Autodesk Fusion 360 part; units mm, degrees
(part 25 of 25)
sketch "Sketch1 (2)" plane through (150, 0, 0) normal (1, 0, 0) x (0, 1, 0) in component "RIght"
  line L0 (64, 0) -> (80, 0)
  line L1 (80, 0) -> (80, 3)
  line L2 (80, 3) -> (64, 3) construction
  line L3 (0, 3) -> (0, 0)
  line L4 (0, 3) -> (0, 160)
  line L5 (0, 160) -> (83, 112.0799)
  line L6 (80, 3) -> (80, 108.0799)
  line L7 (80, 108.0799) -> (83, 108.0799)
  line L8 (83, 108.0799) -> (83, 112.0799)
  circle A0 centre (5.9574, 158.3503) radius 2.9841
  line L9 (4.524, 160.9676) -> (8.9408, 158.4176) construction
  line L10 (8.9408, 158.4176) -> (7.3908, 155.7329) construction
  line L11 (7.3908, 155.7329) -> (2.974, 158.2829) construction
  line L12 (2.974, 158.2829) -> (4.524, 160.9676) construction
  arc A1 (11.1398, 155.3582) -> (0, 157.7854) centre (5.9574, 158.3503) ccw
  line L13 (-5.009, 151.3242) -> (0, 160) construction
  line L14 (11.1398, 155.3582) -> (10.3648, 154.0159) construction
  arc A2 (11.1398, 155.3582) -> (11.7071, 153.2409) centre (12.4821, 154.5832) ccw
  line L15 (64, 3) -> (64, 0)
  line L16 (0, 0) -> (16, 0)
  line L17 (16, 0) -> (16, 3)
  line L18 (80, 0) -> (80, 3)
  line L19 (64, 0) -> (80, 0)
  line L20 (64, 0) -> (64, 3)
  line L21 (48, 3) -> (64, 3)
  line L22 (48, 0) -> (48, 3)
  line L23 (32, 0) -> (48, 0)
  line L24 (32, 0) -> (32, 3)
  line L25 (16, 3) -> (32, 3)
  line L26 (57.0192, 127.0799) -> (58.5192, 129.678)
  line L27 (58.5192, 129.678) -> (67.1795, 124.678)
  line L28 (67.1795, 124.678) -> (65.6795, 122.0799)
  line L29 (0, 145) -> (3, 145)
  line L30 (3, 145) -> (3, 130)
  line L31 (3, 130) -> (0, 130)
  line L32 (80, 68.04) -> (83, 68.04)
  line L33 (83, 68.04) -> (83, 43.04)
  line L34 (83, 43.04) -> (80, 43.04)
  line L35 (83, 55.54) -> (80, 55.54) construction
  dimension "d13" = 60
  dimension "d14" = 160
  dimension "d22" = 3
  dimension "d23" = 4
  dimension "d24" = 3.1
  dimension "d25" = 5.1
  dimension "d26" = 3
  dimension "d45" = 3
  dimension "d46" = 10
  dimension "d47" = 20
  dimension "d54" = 3
  dimension "d55" = 15
  dimension "d56" = 15
  dimension "d60" = 25
  constraint perpendicular L2 L4
  constraint coincident L1.end L2.start
  constraint perpendicular L2 L6
  constraint perpendicular L6 L7
  constraint perpendicular L7 L8
  constraint perpendicular L9 L10
  constraint parallel L9 L11
  constraint parallel L10 L12
  constraint coincident A0 L9.end
  constraint coincident A0 L9.start
  constraint coincident A0 L10.end
  constraint collinear L5 L11
  constraint coincident A0.centre A1.centre
  constraint coincident L5 L14.end
  constraint tangent A1 L14
  constraint perpendicular L5 L13
  constraint perpendicular L5 L14
  constraint tangent A1 L13
  constraint coincident L4 A1.end
  constraint tangent A1 A2
  constraint tangent L5 A2
  constraint coincident L5 A2.end
  constraint coincident L3.start L4.start
  constraint coincident L5 L26.start
  constraint perpendicular L5 L26
  constraint perpendicular L26 L27
  constraint coincident L5 L28.end
  constraint perpendicular L5 L28
  constraint coincident L4 L29.start
  constraint perpendicular L4 L29
  constraint perpendicular L29 L30
  constraint coincident L4 L31.end
  constraint perpendicular L4 L31
  constraint coincident L6 L32.start
  constraint perpendicular L6 L32
  constraint perpendicular L32 L33
  constraint coincident L6 L34.end
  constraint perpendicular L6 L34
  constraint collinear L8 L33
  constraint midpoint L33 L35.start
  constraint midpoint L6 L35.end
  constraint perpendicular L33 L35
  measures "d13" angle of L4 L5
  measures "d14" distance of L3.end L4.end
  measures "d22" distance of L6.end L7.end
  measures "d23" distance of L5.end L7.end
  measures "d24" distance of L9.end L10.end
  measures "d25" distance of L9.start L9.end
  measures "d26" distance of A0 A1
  measures "d45" distance of L26.start L26.end
  measures "d46" distance of L26.end L27.end
  measures "d47" distance of L5.end L28
  measures "d54" distance of L29.start L29.end
  measures "d55" distance of L29.end L30.end
  measures "d56" distance of L4.end L29
  measures "d60" distance of L32.end L33.end
extrude "Extrude1'" add sketch "Sketch1 (2)" along normal blind 3 separate body contours L0 L1 L3 L4 L5 L6 L7 L8 A0 A1 L15 L16 L17 L18 L19 L20 L21 L22 L23 L24 L25 L29 L30 L31 | L6 L32 L33 L34 | L5 L26 L27 L28 | L5 A0 A1 A2 makes body 2 in component "RIght"
sketch "Sketch1 (3)" plane through (0, 0, 0) normal (-1, 0, 0) x (0, -1, 0) in component "Left"
  arc A0 (0, 158.9152) -> (-11.1398, 155.3582) centre (-5.9574, 158.3503) ccw
  arc A1 (-11.7071, 153.2409) -> (-11.1398, 155.3582) centre (-12.4821, 154.5832) ccw
  line L0 (-11.7071, 153.2409) -> (-57.0192, 127.0799)
  circle A2 centre (-5.9574, 158.3503) radius 2.9841
  line L1 (0, 145) -> (0, 158.9152)
  line L2 (-83, 112.0799) -> (-83, 108.0799)
  line L3 (-83, 108.0799) -> (-80, 108.0799)
  line L4 (-80, 43.04) -> (-80, 0)
  line L5 (-80, 0) -> (-64, 0)
  line L6 (-64, 0) -> (-64, 3)
  line L7 (-64, 3) -> (-48, 3)
  line L8 (-48, 3) -> (-48, 0)
  line L9 (-48, 0) -> (-32, 0)
  line L10 (-32, 0) -> (-32, 3)
  line L11 (-32, 3) -> (-16, 3)
  line L12 (-16, 3) -> (-16, 0)
  line L13 (-16, 0) -> (0, 0)
  line L14 (-57.0192, 127.0799) -> (-58.5192, 129.678)
  line L15 (-58.5192, 129.678) -> (-67.1795, 124.678)
  line L16 (-67.1795, 124.678) -> (-65.6795, 122.0799)
  line L17 (-65.6795, 122.0799) -> (-83, 112.0799)
  line L18 (-3, 145) -> (0, 145)
  line L19 (0, 0) -> (0, 130)
  line L20 (0, 130) -> (-3, 130)
  line L21 (-3, 130) -> (-3, 145)
  line L22 (-80, 108.0799) -> (-80, 68.04)
  line L23 (-80, 68.04) -> (-83, 68.04)
  line L24 (-83, 68.04) -> (-83, 43.04)
  line L25 (-83, 43.04) -> (-80, 43.04)
  line L26 (-72.6242, 33.874) -> (-72.6242, 17.226) construction
  line L27 (-72.6242, 17.226) -> (-71.1242, 17.226) construction
  line L28 (-71.1242, 17.226) -> (-71.1242, 33.874) construction
  line L29 (-71.1242, 33.874) -> (-72.6242, 33.874) construction
  line L30 (-74.6242, 35.874) -> (-74.6242, 15.226)
  line L31 (-74.6242, 15.226) -> (-69.1242, 15.226)
  line L32 (-69.1242, 15.226) -> (-69.1242, 35.874)
  line L33 (-69.1242, 35.874) -> (-74.6242, 35.874)
  dimension "d158" = 2
extrude "Extrude1''" add sketch "Sketch1 (3)" along normal blind 3 separate body makes body 3 in component "Left"
sketch "Sketch3" plane through (0, 80, 0) normal (0, 1, 0) x (-1, 0, 0) in component "Back"
  line L0 (-153, 0) -> (-153, 43.04)
  line L1 (3, 43.04) -> (3, 0)
  line L2 (0, 112.0799) -> (0, 108.0799)
  line L3 (-150, 108.0799) -> (-150, 112.0799)
  line L4 (3, 0) -> (-153, 0)
  line L5 (-150, 112.0799) -> (0, 112.0799)
  line L6 (-128.5714, 0) -> (-107.1429, 0)
  line L7 (-107.1429, 0) -> (-107.1429, 3)
  line L8 (-107.1429, 3) -> (-128.5714, 3)
  line L9 (-128.5714, 3) -> (-128.5714, 0)
  line L10 (-85.7143, 0) -> (-64.2857, 0)
  line L11 (-64.2857, 0) -> (-64.2857, 3)
  line L12 (-64.2857, 3) -> (-85.7143, 3)
  line L13 (-85.7143, 3) -> (-85.7143, 0)
  line L14 (-42.8571, 0) -> (-21.4286, 0)
  line L15 (-21.4286, 0) -> (-21.4286, 3)
  line L16 (-21.4286, 3) -> (-42.8571, 3)
  line L17 (-42.8571, 3) -> (-42.8571, 0)
  line L18 (-150, 43.04) -> (-153, 43.04)
  line L19 (-150, 68.04) -> (-150, 43.04)
  line L20 (-150, 68.04) -> (-153, 68.04)
  line L21 (-153, 68.04) -> (-153, 108.0799)
  line L22 (-150, 108.0799) -> (-153, 108.0799)
  line L23 (0, 108.0799) -> (3, 108.0799)
  line L24 (3, 108.0799) -> (3, 68.04)
  line L25 (0, 68.04) -> (3, 68.04)
  line L26 (0, 68.04) -> (0, 43.04)
  line L27 (0, 43.04) -> (3, 43.04)
  circle A0 centre (-6.4309, 71.143) radius 1.5875
  circle A1 centre (-82.7579, 71.143) radius 1.5875
  circle A2 centre (-6.4309, 10.818) radius 1.5875
  circle A3 centre (-82.7579, 10.818) radius 1.5875
  constraint coincident L1.end L4.start
  constraint coincident L0.start L4.end
  constraint coincident L3.end L5.start
  constraint coincident L2.start L5.end
  constraint vertical A1.centre A3.centre
  constraint horizontal A2.centre A3.centre
  constraint equal A0 A3
extrude "Extrude2" add sketch "Sketch3" along normal blind 3 separate body contours L0 L1 L2 L3 L4 L5 L7 L8 L9 L11 L12 L13 L15 L16 L17 L18 L19 L20 L21 L22 L23 L24 L25 L26 L27 makes body 4 in component "Back"
sketch "Sketch1 (4)" plane through (0, 69.282, 120) normal (0, 0.5, 0.866025) x (-1, 0, 0) in component "Fixed Roof"
  line L0 (-150, 4.1599) -> (-153, 4.1599)
  line L1 (-153, 4.1599) -> (-153, -15.8401)
  line L2 (3, 4.1599) -> (3, -15.8401)
  line L3 (0, 4.1599) -> (3, 4.1599)
  line L4 (0, 14.1599) -> (0, 4.1599)
  line L5 (-150, 14.1599) -> (-150, 4.1599)
  line L6 (0, 14.1599) -> (-150, 14.1599)
  line L7 (3, -15.8401) -> (-153, -15.8401)
  constraint coincident L4.start L6.start
  constraint coincident L5.start L6.end
  constraint coincident L2.end L7.start
  constraint coincident L1.end L7.end
extrude "Extrude1'''" add sketch "Sketch1 (4)" along normal blind 3 separate body makes body 5 in component "Fixed Roof"
sketch "Sketch1 (5)" plane through (0, 69.282, 120) normal (0, 0.5, 0.866025) x (-1, 0, 0) in component "Hinged Roof"
  line L0 (-153, 66.4818) -> (-153, 14.1599)
  line L1 (-153, 71.0318) -> (-153, 77)
  line L2 (3, 77) -> (3, 71.0318)
  line L3 (3, 15.1599) -> (-153, 15.1599)
  line L4 (-150, 66.4818) -> (-153, 66.4818)
  line L5 (3, 76.5159) -> (-0.2, 76.5159)
  line L6 (3, 71.5159) -> (-0.2, 71.5159)
  line L7 (-0.2, 76.5159) -> (-0.2, 71.5159) construction
  line L8 (-0.2, 74.0159) -> (3, 74.0159) construction
  line L9 (-0.2, 71.5159) -> (-0.2, 66.4818)
  line L10 (3, 66.4818) -> (-0.2, 66.4818)
  line L11 (0, 77) -> (0, 71.0318) construction
  line L12 (-0.2, 76.5159) -> (-0.2, 78.5159)
  line L13 (-0.2, 78.5159) -> (-149.8, 78.5159)
  line L14 (-75, 15.1599) -> (-75, 78.5159) construction
  line L15 (-153, 66.4818) -> (-149.8, 66.4818)
  line L16 (-149.8, 71.5159) -> (-149.8, 66.4818)
  line L17 (-153, 71.5159) -> (-149.8, 71.5159)
  line L18 (-153, 77) -> (-153, 71.0318)
  line L19 (-153, 76.5159) -> (-149.8, 76.5159)
  line L20 (-149.8, 76.5159) -> (-149.8, 78.5159)
  line L21 (3, 66.4818) -> (3, 14.1599)
  line L22 (-153, 14.1599) -> (-150, 14.1599)
  line L23 (-150, -15.8401) -> (-150, 4.1599)
  line L24 (-150, 4.1599) -> (-153, 4.1599)
  line L25 (-153, 4.1599) -> (-153, -15.8401)
  line L26 (0, 14.1599) -> (-150, 14.1599)
  dimension "d29" = 5
  dimension "d30" = 0.2
  dimension "d31" = 2
  dimension "d34" = 1
  constraint coincident L3.start L21
  constraint coincident L0 L3.end
  constraint perpendicular L0 L3
  constraint coincident L2 L5.start
  constraint perpendicular L2 L5
  constraint coincident L2 L6.start
  constraint perpendicular L2 L6
  constraint midpoint L7 L8.start
  constraint midpoint L2 L8.end
  constraint perpendicular L2 L8
  constraint perpendicular L7 L8
  constraint perpendicular L6 L9
  constraint coincident L10.start L21.start
  constraint perpendicular L9 L10
  constraint perpendicular L5 L12
  constraint perpendicular L12 L13
  constraint midpoint L3 L14.start
  constraint coincident L13 L14.end
  constraint perpendicular L13 L14
  constraint symmetric L2.start L14 L1.end
  constraint symmetric L2.end L14 L1.start
  constraint symmetric L5.start L14 L19.start
  constraint symmetric L5.end L14 L19.end
  constraint symmetric L6.start L14 L17.start
  constraint symmetric L6.end L14 L16.start
  constraint symmetric L9.end L14 L15.end
  constraint symmetric L10.start L14 L0.start
  constraint symmetric L12.end L14 L13.end
  constraint coincident L13.end L20.end
  measures "d29" distance of L5 L6
  measures "d30" distance of L7 L11
  measures "d31" distance of L5.end L12.end
  measures "d34" distance of L3 L26
extrude "Extrude1''''" add sketch "Sketch1 (5)" along normal blind 3 separate body makes body 6 in component "Hinged Roof"
sketch "Sketch4" plane through (0, 3, 0) normal (0, -1, 0) x (1, 0, 0) in component "Front Brace"
  line L0 (0, 130) -> (0, 145)
  line L1 (0, 145) -> (-3, 145)
  line L2 (-3, 145) -> (-3, 130)
  line L3 (-3, 130) -> (0, 130)
  line L4 (150, 145) -> (150, 130)
  line L5 (150, 130) -> (153, 130)
  line L6 (153, 130) -> (153, 145)
  line L7 (153, 145) -> (150, 145)
  line L8 (0, 145) -> (0, 147.5)
  line L9 (0, 147.5) -> (150, 147.5)
  line L10 (150, 147.5) -> (150, 145)
  line L11 (150, 130) -> (150, 127.5)
  line L12 (150, 127.5) -> (0, 127.5)
  line L13 (0, 127.5) -> (0, 130)
  dimension "d59" = 20
  constraint coincident L0.end L1.start
  constraint perpendicular L1 L8
  constraint perpendicular L4 L9
  constraint coincident L4.start L7.end
  constraint perpendicular L7 L10
  constraint coincident L4.end L5.start
  constraint perpendicular L5 L11
  constraint perpendicular L0 L12
  constraint coincident L0.start L3.end
  constraint perpendicular L3 L13
  constraint equal L8 L13
  measures "d59" distance of L9 L12
extrude "Extrude2'" add sketch "Sketch4" along normal blind 3 separate body makes body 7 in component "Front Brace"
sketch "Sketch3 (2)" plane through (-3, 0, 0) normal (-1, 0, 0) x (0, -1, 0) in component "Left"
  arc A0 (0, 158.9152) -> (-11.1398, 155.3582) centre (-5.9574, 158.3503) ccw
  arc A1 (-11.7071, 153.2409) -> (-11.1398, 155.3582) centre (-12.4821, 154.5832) ccw
  circle A2 centre (-18.9112, 127.6636) radius 1.75
  circle A3 centre (-18.9112, 127.6636) radius 1.75
  line L0 (-16.6612, 120.2136) -> (-26.6612, 120.2136) construction
  line L1 (-26.6612, 120.2136) -> (-26.6612, 117.7136) construction
  line L2 (-26.6612, 117.7136) -> (-16.6612, 117.7136) construction
  line L3 (-16.6612, 117.7136) -> (-16.6612, 120.2136) construction
  line L4 (-27.6612, 116.7136) -> (-15.6612, 116.7136)
  line L5 (-15.6612, 116.7136) -> (-15.6612, 121.2136)
  line L6 (-15.6612, 121.2136) -> (-27.6612, 121.2136)
  line L7 (-27.6612, 121.2136) -> (-27.6612, 116.7136)
  circle A4 centre (-51.5891, 107.0301) radius 3
  line L8 (-11.7071, 153.2409) -> (-57.0192, 127.0799)
  circle A5 centre (-5.9574, 158.3503) radius 2.9841
  line L9 (-83, 112.0799) -> (-83, 108.0799)
  line L10 (-83, 108.0799) -> (-80, 108.0799)
  line L11 (-80, 43.04) -> (-80, 0)
  line L12 (-80, 0) -> (-64, 0)
  line L13 (-64, 0) -> (-64, 3)
  line L14 (-64, 3) -> (-48, 3)
  line L15 (-48, 3) -> (-48, 0)
  line L16 (-48, 0) -> (-32, 0)
  line L17 (-32, 0) -> (-32, 3)
  line L18 (-32, 3) -> (-16, 3)
  line L19 (-16, 3) -> (-16, 0)
  line L20 (-16, 0) -> (0, 0)
  line L21 (0, 145) -> (0, 158.9152)
  line L22 (-57.0192, 127.0799) -> (-58.5192, 129.678)
  line L23 (-58.5192, 129.678) -> (-67.1795, 124.678)
  line L24 (-67.1795, 124.678) -> (-65.6795, 122.0799)
  line L25 (-65.6795, 122.0799) -> (-83, 112.0799)
  line L26 (0, 0) -> (0, 130)
  line L27 (0, 130) -> (-3, 130)
  line L28 (-3, 130) -> (-3, 145)
  line L29 (-3, 145) -> (0, 145)
  line L30 (-80, 108.0799) -> (-80, 68.04)
  line L31 (-80, 68.04) -> (-83, 68.04)
  line L32 (-83, 68.04) -> (-83, 43.04)
  line L33 (-83, 43.04) -> (-80, 43.04)
  line L34 (-12.7904, 87.8786) -> (-15.2904, 87.8786)
  arc A6 (-12.7904, 85.8786) -> (-12.7904, 87.8786) centre (-12.7904, 86.8786) ccw
  line L35 (-15.2904, 85.8786) -> (-12.7904, 85.8786)
  arc A7 (-15.2904, 87.8786) -> (-15.2904, 85.8786) centre (-15.2904, 86.8786) ccw
  line L36 (-12.7904, 63.8786) -> (-15.2904, 63.8786)
  arc A8 (-12.7904, 61.8786) -> (-12.7904, 63.8786) centre (-12.7904, 62.8786) ccw
  line L37 (-15.2904, 61.8786) -> (-12.7904, 61.8786)
  arc A9 (-15.2904, 63.8786) -> (-15.2904, 61.8786) centre (-15.2904, 62.8786) ccw
  line L38 (-37.2904, 63.8786) -> (-39.7904, 63.8786)
  arc A10 (-39.7904, 63.8786) -> (-39.7904, 61.8786) centre (-39.7904, 62.8786) ccw
  line L39 (-39.7904, 61.8786) -> (-37.2904, 61.8786)
  arc A11 (-37.2904, 61.8786) -> (-37.2904, 63.8786) centre (-37.2904, 62.8786) ccw
  arc A12 (-37.2904, 85.8786) -> (-37.2904, 87.8786) centre (-37.2904, 86.8786) ccw
  line L40 (-37.2904, 87.8786) -> (-39.7904, 87.8786)
  arc A13 (-39.7904, 87.8786) -> (-39.7904, 85.8786) centre (-39.7904, 86.8786) ccw
  line L41 (-39.7904, 85.8786) -> (-37.2904, 85.8786)
  line L42 (-31.1904, 88.3786) -> (-21.3904, 88.3786) construction
  line L43 (-21.3904, 88.3786) -> (-21.3904, 85.7786) construction
  line L44 (-21.3904, 85.7786) -> (-31.1904, 85.7786) construction
  line L45 (-31.1904, 85.7786) -> (-31.1904, 88.3786) construction
  line L46 (-20.8904, 85.2786) -> (-31.6904, 85.2786)
  line L47 (-31.6904, 85.2786) -> (-31.6904, 88.8786)
  line L48 (-31.6904, 88.8786) -> (-20.8904, 88.8786)
  line L49 (-20.8904, 88.8786) -> (-20.8904, 85.2786)
  line L50 (-74.6242, 35.874) -> (-69.1242, 35.874)
  line L51 (-69.1242, 35.874) -> (-69.1242, 15.226)
  line L52 (-69.1242, 15.226) -> (-74.6242, 15.226)
  line L53 (-74.6242, 15.226) -> (-74.6242, 35.874)
  line L54 (-26.6612, 120.2136) -> (-16.6612, 117.7136) construction
  line L55 (-21.3904, 88.3786) -> (-31.1904, 85.7786) construction
  line L56 (-26.2904, 87.0786) -> (-51.5891, 107.0301) construction
  line L57 (-51.5891, 107.0301) -> (-21.6612, 118.9636) construction
  dimension "d35" = 1
  dimension "d36" = 6
  dimension "d157" = -0.5
  dimension "d159" = 60
  constraint coincident L0.end L1.start
  constraint coincident L2.end L3.start
  constraint coincident L42.end L43.start
  constraint coincident L44.end L45.start
  constraint midpoint L55 L56.start
  constraint coincident A4.centre L56.end
  constraint midpoint L54 L57.end
  constraint equal L56 L57
  measures "d36" diameter of A4
  measures "d159" angle of L56 L57
extrude "Extrude2''" cut sketch "Sketch3 (2)" against normal up to surface (3 mm away) contours A2 A3 | L4 L5 L6 L7 | A4 | L34 A6 L35 A7 | L36 A8 L37 A9 | L38 A10 L39 A11 | A12 L40 A13 L41 | L46 L47 L48 L49 bodies 3 in component "Left"
sketch "Sketch2" plane through (153, 0, 0) normal (1, 0, 0) x (0, 1, 0) in component "RIght"
  circle A0 centre (5.9574, 158.3503) radius 2.9841
  line L0 (80, 68.04) -> (80, 108.0799)
  line L1 (80, 108.0799) -> (83, 108.0799)
  line L2 (83, 108.0799) -> (83, 112.0799)
  line L3 (83, 112.0799) -> (65.6795, 122.0799)
  line L4 (65.6795, 122.0799) -> (67.1795, 124.678)
  line L5 (67.1795, 124.678) -> (58.5192, 129.678)
  line L6 (58.5192, 129.678) -> (57.0192, 127.0799)
  line L7 (57.0192, 127.0799) -> (11.7071, 153.2409)
  arc A1 (11.1398, 155.3582) -> (11.7071, 153.2409) centre (12.4821, 154.5832) ccw
  arc A2 (11.1398, 155.3582) -> (0, 158.9152) centre (5.9574, 158.3503) ccw
  line L8 (0, 158.9152) -> (0, 145)
  line L9 (0, 145) -> (3, 145)
  line L10 (3, 145) -> (3, 130)
  line L11 (3, 130) -> (0, 130)
  line L12 (0, 130) -> (0, 0)
  line L13 (0, 0) -> (16, 0)
  line L14 (16, 0) -> (16, 3)
  line L15 (16, 3) -> (32, 3)
  line L16 (32, 3) -> (32, 0)
  line L17 (32, 0) -> (48, 0)
  line L18 (48, 0) -> (48, 3)
  line L19 (48, 3) -> (64, 3)
  line L20 (64, 3) -> (64, 0)
  line L21 (64, 0) -> (80, 0)
  line L22 (80, 0) -> (80, 43.04)
  line L23 (80, 43.04) -> (83, 43.04)
  line L24 (83, 43.04) -> (83, 68.04)
  line L25 (83, 68.04) -> (80, 68.04)
  arc A3 (10.3278, 35.6711) -> (11.6278, 35.6711) centre (10.9778, 34.9111) ccw
  arc A4 (11.6278, 6.8512) -> (10.3278, 6.8512) centre (10.9778, 7.6111) ccw
  arc A5 (10.3278, 6.8512) -> (11.6278, 6.8512) centre (10.9778, 7.6111) ccw
  arc A6 (11.6278, 35.6711) -> (10.3278, 35.6711) centre (10.9778, 34.9111) ccw
  line L26 (16.8528, 26.6361) -> (16.8528, 10.0111) construction
  line L27 (16.8528, 32.5111) -> (16.8528, 26.6361) construction
  line L28 (10.9778, 32.5111) -> (16.8528, 32.5111) construction
  line L29 (5.1028, 32.5111) -> (10.9778, 32.5111) construction
  line L30 (5.1028, 26.6361) -> (5.1028, 32.5111) construction
  line L31 (5.1028, 10.0111) -> (5.1028, 26.6361) construction
  line L32 (5.1028, 10.0111) -> (16.8528, 10.0111) construction
  line L33 (4.9028, 9.8111) -> (17.0528, 9.8111)
  line L34 (17.0528, 26.6361) -> (17.0528, 9.8111)
  line L35 (17.0528, 32.7111) -> (17.0528, 26.6361)
  line L36 (10.9778, 32.7111) -> (17.0528, 32.7111)
  line L37 (4.9028, 32.7111) -> (10.9778, 32.7111)
  line L38 (4.9028, 26.6361) -> (4.9028, 32.7111)
  line L39 (4.9028, 9.8111) -> (4.9028, 26.6361)
  dimension "d94" = 0.2
  constraint coincident A4.start A5.end
  constraint coincident A4.centre A5.centre
  constraint coincident A3.end A6.start
  constraint coincident A3.centre A6.centre
  constraint coincident A3.start A6.end
  constraint coincident A4.end A5.start
extrude "Extrude2'''" cut sketch "Sketch2" against normal up to surface (3 mm away) contours A3 A6 | A4 A5 | L33 L34 L35 L36 L37 L38 L39 bodies 2 in component "RIght"
sketch "Sketch13" plane through (0, 70.782, 122.5981) normal (0, 0.5, 0.866025) x (-1, 0, 0)
  line L0 (0, 14.1599) -> (-150, 14.1599)
  line L1 (-150, 14.1599) -> (-150, 4.1599)
  line L2 (-150, 4.1599) -> (-153, 4.1599)
  line L3 (-153, 4.1599) -> (-153, -15.8401)
  line L4 (-153, -15.8401) -> (3, -15.8401)
  line L5 (3, -15.8401) -> (3, 4.1599)
  line L6 (3, 4.1599) -> (0, 4.1599)
  line L7 (0, 4.1599) -> (0, 14.1599)
sketch "Sketch14" plane through (-0.0564, 70.7234, 122.6319) normal (0, 0.5, 0.866025) x (-1, 0, 0)
  line L0 (-153.0564, 15.0922) -> (2.9436, 15.0922)
  line L1 (2.9436, 15.0922) -> (2.9436, 66.4141)
  line L2 (2.9436, 66.4141) -> (-0.2564, 66.4141)
  line L3 (-0.2564, 66.4141) -> (-0.2564, 71.4482)
  line L4 (-0.2564, 71.4482) -> (2.9436, 71.4482)
  line L5 (2.9436, 71.4482) -> (2.9436, 76.4482)
  line L6 (2.9436, 76.4482) -> (-0.2564, 76.4482)
  line L7 (-0.2564, 76.4482) -> (-0.2564, 78.4482)
  line L8 (-0.2564, 78.4482) -> (-149.8564, 78.4482)
  line L9 (-149.8564, 78.4482) -> (-149.8564, 76.4482)
  line L10 (-149.8564, 76.4482) -> (-153.0564, 76.4482)
  line L11 (-153.0564, 76.4482) -> (-153.0564, 71.4482)
  line L12 (-153.0564, 71.4482) -> (-149.8564, 71.4482)
  line L13 (-149.8564, 71.4482) -> (-149.8564, 66.4141)
  line L14 (-149.8564, 66.4141) -> (-153.0564, 66.4141)
  line L15 (-153.0564, 66.4141) -> (-153.0564, 15.0922)
sketch "Sketch15" plane through (153, 0, 0) normal (1, 0, 0) x (0, 1, 0)
  circle A0 centre (10.9778, 7.6111) radius 1
  circle A1 centre (10.9778, 34.9111) radius 1
  line L0 (4.9028, 9.8111) -> (4.9028, 32.7111)
  line L1 (4.9028, 32.7111) -> (17.0528, 32.7111)
  line L2 (17.0528, 32.7111) -> (17.0528, 9.8111)
  line L3 (17.0528, 9.8111) -> (4.9028, 9.8111)
  circle A2 centre (5.9574, 158.3503) radius 2.9841
  line L4 (80, 68.04) -> (80, 108.0799)
  line L5 (80, 108.0799) -> (83, 108.0799)
  line L6 (83, 108.0799) -> (83, 112.0799)
  line L7 (83, 112.0799) -> (65.6795, 122.0799)
  line L8 (65.6795, 122.0799) -> (67.1795, 124.678)
  line L9 (67.1795, 124.678) -> (58.5192, 129.678)
  line L10 (58.5192, 129.678) -> (57.0192, 127.0799)
  line L11 (57.0192, 127.0799) -> (11.7071, 153.2409)
  arc A3 (11.1398, 155.3582) -> (11.7071, 153.2409) centre (12.4821, 154.5832) ccw
  arc A4 (11.1398, 155.3582) -> (0, 158.9152) centre (5.9574, 158.3503) ccw
  line L12 (0, 158.9152) -> (0, 145)
  line L13 (0, 145) -> (3, 145)
  line L14 (3, 145) -> (3, 130)
  line L15 (3, 130) -> (0, 130)
  line L16 (0, 130) -> (0, 0)
  line L17 (0, 0) -> (16, 0)
  line L18 (16, 0) -> (16, 3)
  line L19 (16, 3) -> (32, 3)
  line L20 (32, 3) -> (32, 0)
  line L21 (32, 0) -> (48, 0)
  line L22 (48, 0) -> (48, 3)
  line L23 (48, 3) -> (64, 3)
  line L24 (64, 3) -> (64, 0)
  line L25 (64, 0) -> (80, 0)
  line L26 (80, 0) -> (80, 43.04)
  line L27 (80, 43.04) -> (83, 43.04)
  line L28 (83, 43.04) -> (83, 68.04)
  line L29 (83, 68.04) -> (80, 68.04)
sketch "Sketch16" plane through (0, 0, 0) normal (1, 0, 0) x (0, 1, 0)
  circle A0 centre (18.9112, 127.6636) radius 1.75
  line L0 (15.6612, 121.2136) -> (27.6612, 121.2136)
  line L1 (27.6612, 121.2136) -> (27.6612, 116.7136)
  line L2 (27.6612, 116.7136) -> (15.6612, 116.7136)
  line L3 (15.6612, 116.7136) -> (15.6612, 121.2136)
  circle A1 centre (51.5891, 107.0301) radius 3
  circle A2 centre (5.9574, 158.3503) radius 2.9841
  line L4 (57.0192, 127.0799) -> (11.7071, 153.2409)
  arc A3 (11.1398, 155.3582) -> (11.7071, 153.2409) centre (12.4821, 154.5832) ccw
  arc A4 (11.1398, 155.3582) -> (0, 158.9152) centre (5.9574, 158.3503) ccw
  line L5 (0, 158.9152) -> (0, 145)
  line L6 (0, 145) -> (3, 145)
  line L7 (3, 145) -> (3, 130)
  line L8 (3, 130) -> (0, 130)
  line L9 (0, 130) -> (0, 0)
  line L10 (0, 0) -> (16, 0)
  line L11 (16, 0) -> (16, 3)
  line L12 (16, 3) -> (32, 3)
  line L13 (32, 3) -> (32, 0)
  line L14 (32, 0) -> (48, 0)
  line L15 (48, 0) -> (48, 3)
  line L16 (48, 3) -> (64, 3)
  line L17 (64, 3) -> (64, 0)
  line L18 (64, 0) -> (80, 0)
  line L19 (80, 0) -> (80, 43.04)
  line L20 (80, 43.04) -> (83, 43.04)
  line L21 (83, 43.04) -> (83, 68.04)
  line L22 (83, 68.04) -> (80, 68.04)
  line L23 (80, 68.04) -> (80, 108.0799)
  line L24 (80, 108.0799) -> (83, 108.0799)
  line L25 (83, 108.0799) -> (83, 112.0799)
  line L26 (83, 112.0799) -> (65.6795, 122.0799)
  line L27 (65.6795, 122.0799) -> (67.1795, 124.678)
  line L28 (67.1795, 124.678) -> (58.5192, 129.678)
  line L29 (58.5192, 129.678) -> (57.0192, 127.0799)
  line L30 (39.7904, 61.8786) -> (37.2904, 61.8786)
  arc A5 (37.2904, 63.8786) -> (37.2904, 61.8786) centre (37.2904, 62.8786) ccw
  line L31 (37.2904, 63.8786) -> (39.7904, 63.8786)
  arc A6 (39.7904, 61.8786) -> (39.7904, 63.8786) centre (39.7904, 62.8786) ccw
  arc A7 (39.7904, 85.8786) -> (39.7904, 87.8786) centre (39.7904, 86.8786) ccw
  line L32 (39.7904, 85.8786) -> (37.2904, 85.8786)
  arc A8 (37.2904, 87.8786) -> (37.2904, 85.8786) centre (37.2904, 86.8786) ccw
  line L33 (37.2904, 87.8786) -> (39.7904, 87.8786)
  line L34 (12.7904, 63.8786) -> (15.2904, 63.8786)
  arc A9 (15.2904, 61.8786) -> (15.2904, 63.8786) centre (15.2904, 62.8786) ccw
  line L35 (15.2904, 61.8786) -> (12.7904, 61.8786)
  arc A10 (12.7904, 63.8786) -> (12.7904, 61.8786) centre (12.7904, 62.8786) ccw
  line L36 (12.7904, 87.8786) -> (15.2904, 87.8786)
  arc A11 (15.2904, 85.8786) -> (15.2904, 87.8786) centre (15.2904, 86.8786) ccw
  line L37 (15.2904, 85.8786) -> (12.7904, 85.8786)
  arc A12 (12.7904, 87.8786) -> (12.7904, 85.8786) centre (12.7904, 86.8786) ccw
  line L38 (20.8904, 85.2786) -> (20.8904, 88.8786)
  line L39 (20.8904, 88.8786) -> (31.6904, 88.8786)
  line L40 (31.6904, 88.8786) -> (31.6904, 85.2786)
  line L41 (31.6904, 85.2786) -> (20.8904, 85.2786)
  line L42 (69.1242, 35.874) -> (74.6242, 35.874)
  line L43 (74.6242, 35.874) -> (74.6242, 15.226)
  line L44 (74.6242, 15.226) -> (69.1242, 15.226)
  line L45 (69.1242, 15.226) -> (69.1242, 35.874)
sketch "Sketch17" plane through (0, 0, 0) normal (0, -1, 0) x (1, 0, 0)
  line L0 (150, 130) -> (153, 130)
  line L1 (153, 130) -> (153, 145)
  line L2 (153, 145) -> (150, 145)
  line L3 (150, 145) -> (150, 147.5)
  line L4 (150, 147.5) -> (0, 147.5)
  line L5 (0, 147.5) -> (0, 145)
  line L6 (0, 145) -> (-3, 145)
  line L7 (-3, 145) -> (-3, 130)
  line L8 (-3, 130) -> (0, 130)
  line L9 (0, 130) -> (0, 127.5)
  line L10 (0, 127.5) -> (150, 127.5)
  line L11 (150, 127.5) -> (150, 130)
sketch "Sketch18" plane through (0, 83, 0) normal (0, 1, 0) x (-1, 0, 0)
  line L0 (0, 68.04) -> (3, 68.04)
  line L1 (3, 68.04) -> (3, 108.0799)
  line L2 (3, 108.0799) -> (0, 108.0799)
  line L3 (0, 108.0799) -> (0, 112.0799)
  line L4 (0, 112.0799) -> (-150, 112.0799)
  line L5 (-150, 112.0799) -> (-150, 108.0799)
  line L6 (-150, 108.0799) -> (-153, 108.0799)
  line L7 (-153, 108.0799) -> (-153, 68.04)
  line L8 (-153, 68.04) -> (-150, 68.04)
  line L9 (-150, 68.04) -> (-150, 43.04)
  line L10 (-150, 43.04) -> (-153, 43.04)
  line L11 (-153, 43.04) -> (-153, 0)
  line L12 (-153, 0) -> (-128.5714, 0)
  line L13 (-128.5714, 0) -> (-128.5714, 3)
  line L14 (-128.5714, 3) -> (-107.1429, 3)
  line L15 (-107.1429, 3) -> (-107.1429, 0)
  line L16 (-107.1429, 0) -> (-85.7143, 0)
  line L17 (-85.7143, 0) -> (-85.7143, 3)
  line L18 (-85.7143, 3) -> (-64.2857, 3)
  line L19 (-64.2857, 3) -> (-64.2857, 0)
  line L20 (-64.2857, 0) -> (-42.8571, 0)
  line L21 (-42.8571, 0) -> (-42.8571, 3)
  line L22 (-42.8571, 3) -> (-21.4286, 3)
  line L23 (-21.4286, 3) -> (-21.4286, 0)
  line L24 (-21.4286, 0) -> (3, 0)
  line L25 (3, 0) -> (3, 43.04)
  line L26 (3, 43.04) -> (0, 43.04)
  line L27 (0, 43.04) -> (0, 68.04)
  circle A0 centre (-6.4309, 10.818) radius 1.5875
  circle A1 centre (-82.7579, 10.818) radius 1.5875
  circle A2 centre (-6.4309, 71.143) radius 1.5875
  circle A3 centre (-82.7579, 71.143) radius 1.5875
sketch "Sketch19" plane through (0, 0, 3) normal (0, 0, 1) x (-1, 0, 0)
  line L0 (-150, -64) -> (-150, -80)
  line L1 (-150, -80) -> (-128.5714, -80)
  line L2 (-128.5714, -80) -> (-128.5714, -83)
  line L3 (-128.5714, -83) -> (-107.1429, -83)
  line L4 (-107.1429, -83) -> (-107.1429, -80)
  line L5 (-107.1429, -80) -> (-85.7143, -80)
  line L6 (-85.7143, -80) -> (-85.7143, -83)
  line L7 (-85.7143, -83) -> (-64.2857, -83)
  line L8 (-64.2857, -83) -> (-64.2857, -80)
  line L9 (-64.2857, -80) -> (-42.8571, -80)
  line L10 (-42.8571, -80) -> (-42.8571, -83)
  line L11 (-42.8571, -83) -> (-21.4286, -83)
  line L12 (-21.4286, -83) -> (-21.4286, -80)
  line L13 (-21.4286, -80) -> (0, -80)
  line L14 (0, -80) -> (0, -64)
  line L15 (0, -64) -> (3, -64)
  line L16 (3, -64) -> (3, -48)
  line L17 (3, -48) -> (0, -48)
  line L18 (0, -48) -> (0, -32)
  line L19 (0, -32) -> (3, -32)
  line L20 (3, -32) -> (3, -16)
  line L21 (3, -16) -> (0, -16)
  line L22 (0, -16) -> (0, 0)
  line L23 (0, 0) -> (-150, 0)
  line L24 (-150, 0) -> (-150, -16)
  line L25 (-150, -16) -> (-153, -16)
  line L26 (-153, -16) -> (-153, -32)
  line L27 (-153, -32) -> (-150, -32)
  line L28 (-150, -32) -> (-150, -48)
  line L29 (-150, -48) -> (-153, -48)
  line L30 (-153, -48) -> (-153, -64)
  line L31 (-153, -64) -> (-150, -64)
component "Base" placed x (1, 0, 0) y (0, 1, 0) z (0, 0, 1) at (0, 0, 0)
component "RIght" placed x (1, 0, 0) y (0, 1, 0) z (0, 0, 1) at (0, 0, 0)
component "Left" placed x (1, 0, 0) y (0, 1, 0) z (0, 0, 1) at (0, 0, 0)
component "Back" placed x (1, 0, 0) y (0, 1, 0) z (0, 0, 1) at (0, 0, 0)
component "Fixed Roof" placed x (1, 0, 0) y (0, 1, 0) z (0, 0, 1) at (0, 0, 0)
component "Hinged Roof" placed x (1, 0, 0) y (0, 1, 0) z (0, 0, 1) at (0, 0, 0)
component "Front Brace" placed x (1, 0, 0) y (0, 1, 0) z (0, 0, 1) at (0, 0, 0)

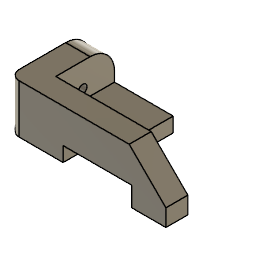
design "mount"
part number: 2026-05-03-20-23-12-046
Autodesk Fusion 360 part; units mm, degrees
sketch "Sketch20" plane through (0, 0, 0) normal (0, 0, 1) x (1, 0, 0)
  line L0 (0, 0) -> (-32, 0)
  line L1 (0, 0) -> (0, 4.5)
  line L2 (0, 4.5) -> (-27, 4.5)
  line L3 (-27, 16.5) -> (-27, 4.5)
  line L4 (-32, 0) -> (-32, 16.5)
  line L5 (-27, 16.5) -> (-32, 16.5)
  dimension "d60" = 32
  dimension "d61" = 4.5
  dimension "d62" = 27
  dimension "d66" = 12
  constraint coincident L0.start L1.start
  constraint horizontal L0
  constraint perpendicular L0 L1
  constraint perpendicular L1 L2
  constraint perpendicular L0 L4
  measures "d60" distance of L0.start L0.end
  measures "d61" distance of L0.start L1.end
  measures "d62" distance of L1.end L2.end
  measures "d66" distance of L2.end L3.start
extrude "Extrude12" add sketch "Sketch20" along normal blind 10 makes body 1
sketch "Sketch21" plane through (0, 4.5, 0) normal (0, 1, 0) x (-1, 0, 0)
  line L0 (0, 0) -> (27, 0)
  line L1 (27, 0) -> (27, 10)
  line L2 (27, 10) -> (0, 10)
  line L3 (0, 10) -> (0, 0)
  line L4 (27, 0) -> (21, 0)
  line L5 (27, 3) -> (27, 0)
  line L6 (21, 0) -> (7, 0)
  line L7 (7, 0) -> (7, 3)
  line L8 (7, 3) -> (21, 3)
  line L9 (21, 3) -> (21, 0)
  dimension "d69" = 6
  dimension "d71" = 27
  dimension "d72" = 14
  dimension "d73" = 3
  constraint coincident L0.end L1.start
  constraint perpendicular L1 L4
  constraint coincident L1 L5.start
  constraint parallel L0 L6
  constraint perpendicular L6 L7
  constraint perpendicular L7 L8
  measures "d69" distance of L0.end L4.end
  measures "d71" distance of L0.start L0.end
  measures "d72" distance of L4.end L6.end
  measures "d73" distance of L6.end L7.end
extrude "Extrude13" cut sketch "Sketch21" against normal blind 7 contours L0 L6 L7 L8 L9 bodies 1
sketch "Sketch22" plane through (0, 0, 0) normal (0, 0, 1) x (1, 0, 0)
  line L0 (-27, 4.5) -> (-15, 4.5)
  line L1 (-27, 16.5) -> (-27, 4.5)
  line L2 (-15, 4.5) -> (-15, 16.5)
  line L3 (-15, 16.5) -> (-27, 16.5)
  dimension "d76" = 12
  dimension "d77" = 12
  constraint horizontal L0
  constraint perpendicular L0 L2
  measures "d76" distance of L0.start L0.end
  measures "d77" distance of L0.end L2.end
extrude "Extrude14" add sketch "Sketch22" along normal blind 3 separate body makes body 2
extrude "Extrude15" add 1 faces at (-2.3333, 1.5, 0) along direction (0, 0, -1) blind 1 on bodies 1 bodies 1
sketch "Sketch23" plane through (-32, 0, 0) normal (-1, 0, 0) x (0, -1, 0)
  line L0 (-16.5, 0) -> (0, 0)
  line L1 (0, 0) -> (0, 10)
  line L2 (0, 10) -> (-16.5, 10)
  line L3 (-16.5, 10) -> (-16.5, 0)
  circle A0 centre (-10, 5) radius 0.8695
  dimension "d82" = 1.739
  measures "d82" diameter of A0
extrude "Extrude16" cut sketch "Sketch23" against normal blind 10.5 contours A0 bodies 1
fillet "Fillet3" radius 5 1 edges at (-29.5, 16.5, 10) on bodies 1
chamfer "Chamfer4" distance 1 angle 45 1 edges at (-32, 8.25, 0) on bodies 1
chamfer "Chamfer5" distance 7.5 angle 45 1 edges at (0, 2.25, 10) on bodies 1
fillet "Fillet4" radius 2 1 edges at (-32, 0, 5.5) on bodies 1

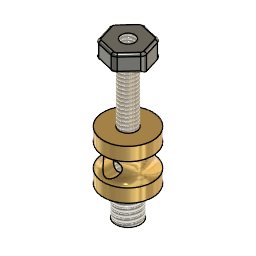
design "push rod connector"
Autodesk Fusion 360 part; units mm, degrees
sketch "Sketch1" plane through (0, 0, 0) normal (0, 0, 1) x (1, 0, 0) in component "push rod connector"
  circle A0 centre (0, 0) radius 2.5
  circle A1 centre (0, 0) radius 1.3
  dimension "d1" = 5
  dimension "d25" = 2.6
  constraint coincident A0.centre A1.centre
  measures "d1" diameter of A0
  measures "d25" diameter of A1
extrude "Extrude1" add sketch "Sketch1" along normal blind 5 contours A0 | A1 makes body 1 in component "push rod connector"
sketch "Sketch2" plane through (0, 0, 5) normal (0, 0, 1) x (-1, 0, 0) in component "push rod connector"
  circle A0 centre (0, 0) radius 2.5
  circle A1 centre (0, 0) radius 0.875
  dimension "d4" = 1.75
  constraint coincident A0.centre A1.centre
  measures "d4" diameter of A1
extrude "Extrude2" add sketch "Sketch2" along normal blind 6 contours A1 bodies 1 in component "push rod connector"
sketch "Sketch6" plane through (0, 0, 0) normal (0, 1, 0) x (1, 0, 0) in component "push rod connector"
  circle A0 centre (0, -2.5) radius 0.95
  line L0 (-2.5, -5) -> (2.5, -5) construction
  line L1 (-2.5, 0) -> (2.5, 0) construction
  line L2 (0, -5) -> (0, 0) construction
  dimension "d9" = 1.9
  constraint midpoint L0 L2.start
  constraint coincident L2.end origin
  constraint midpoint A0.centre L2
  measures "d9" diameter of A0
extrude "Extrude3" cut sketch "Sketch6" against normal through all and the other way through all bodies 1 in component "push rod connector"
sketch "Sketch3" plane through (0, 0, 0) normal (0, 1, 0) x (1, 0, 0)
  line L0 (-2.5, 0) -> (2.5, 0) construction
  line L1 (-2.5, -5) -> (2.5, -5) construction
  line L2 (2.5, -5) -> (2.5, 0)
  arc A0 (2.5, -1.3467) -> (2.5, -3.6533) centre (3.1, -2.5) ccw
  line L3 (3.1, -2.5) -> (2.5, -2.5) construction
  dimension "d23" = 0.6
  dimension "d24" = 1.3
  constraint coincident L1.end L2.start
  constraint coincident L0.end L2.end
  constraint coincident L2 A0.end
  constraint coincident L2 A0.start
  constraint coincident A0.centre L3.start
  constraint coincident L2 L3.end
  constraint perpendicular L2 L3
  constraint midpoint L2 L3.end
  measures "d23" distance of A0.centre L3.end
  measures "d24" radius of A0
revolve "Revolve1" cut sketch "Sketch3" angle 360 about axis through (0, 0, 1.75) along (0, 0, 1) bodies 1 in component "push rod connector"
extrude "Extrude5" cut sketch "Sketch1" along normal blind 3.7 contours A1 bodies 1 in component "push rod connector"
sketch "Sketch1 (2)" plane through (0, 0, 0) normal (0, 0, -1) x (1, 0, 0) in component "grub screw"
  circle A0 centre (0, 0) radius 1.3
  circle A1 centre (0, 0) radius 2.5
extrude "Extrude1'" add sketch "Sketch1 (2)" along normal blind 3 separate body contours A0 makes body 2 in component "grub screw"
chamfer "Chamfer1" distance 0.7 angle 45 1 edges at (-1.212, 0.4701, 0) on bodies 2 in component "grub screw"
sketch "Sketch2 (2)" plane through (0, 0, -3) normal (0, 0, -1) x (1, 0, 0) in component "grub screw"
  circle A0 centre (0, 0) radius 1.3
  line L0 (0.6928, 0.4) -> (0, 0.8)
  line L1 (0, 0.8) -> (-0.6928, 0.4)
  line L2 (-0.6928, 0.4) -> (-0.6928, -0.4)
  line L3 (-0.6928, -0.4) -> (0, -0.8)
  line L4 (0, -0.8) -> (0.6928, -0.4)
  line L5 (0.6928, -0.4) -> (0.6928, 0.4)
  dimension "d29" = 0.8
  constraint coincident A0.centre origin
  constraint vertical L5
  measures "d29" distance of L0.start A0.centre
extrude "Extrude2'" cut sketch "Sketch2 (2)" against normal blind 1.478 contours L0 L1 L2 L3 L4 L5 bodies 2 in component "grub screw"
sketch "Sketch1 (3)" plane through (0, 0, 11) normal (0, 0, 1) x (-1, 0, 0) in component "hex nut"
  circle A0 centre (0, 0) radius 0.875
  line L0 (0.6569, -2.1537) -> (2.1936, -0.5079)
  line L1 (2.1936, -0.5079) -> (1.5367, 1.6458)
  line L2 (1.5367, 1.6458) -> (-0.6569, 2.1537)
  line L3 (-0.6569, 2.1537) -> (-2.1936, 0.5079)
  line L4 (-2.1936, 0.5079) -> (-1.5367, -1.6458)
  line L5 (-1.5367, -1.6458) -> (0.6569, -2.1537)
  dimension "d32" = 1.95
  constraint coincident A0.centre origin
  measures "d32" distance of A0.centre L5
extrude "Extrude1''" add sketch "Sketch1 (3)" along normal blind 1.7 separate body makes body 3 in component "hex nut"
fillet "Fillet1" radius 0.494 6 edges at (0.6569, -2.1537, 11.85) (-1.5367, -1.6458, 11.85) (-2.1936, 0.5079, 11.85) (-0.6569, 2.1537, 11.85) (1.5367, 1.6458, 11.85) (2.1936, -0.5079, 11.85) on bodies 3 in component "hex nut"
fillet "Fillet1" radius 0.222 11 edges at (1.4253, -1.3308, 12.7) (-0.4399, -1.8997, 12.7) (-1.8652, -0.5689, 12.7) (-1.4253, 1.3308, 12.7) (0.4399, 1.8997, 12.7) (0.4399, 1.8997, 11) (-1.4253, 1.3308, 11) (-1.8652, -0.5689, 11) (-0.4399, -1.8997, 11) (1.4253, -1.3308, 11) (1.8652, 0.5689, 12.7) on bodies 3 in component "hex nut"
thread "Thread1" "ISO Metric profile 1.8 M1.8x0.35 6g" major diameter 1.7385 minor diameter 1.3386 pitch 0.35 angle 60 resizes the face on face at (-0.8739, 0.0436, 9) on bodies 1 in component "push rod connector"
thread "Thread1'" "ISO Metric profile 2.6 M2.6x0.45 6g" major diameter 2.53 minor diameter 2.0162 pitch 0.45 angle 60 resizes the face on face at (1.2935, 0.1294, -1.4667) on bodies 2 in component "grub screw"
thread "Thread2" "ISO Metric profile 2.5 M2.5x0.45 6H" major diameter 2.58 minor diameter 2.0755 pitch 0.45 angle 60 resizes the face on face at (-1.0349, -0.7868, 2.0472) on bodies 1 in component "push rod connector"
thread "Thread1''" "ISO Metric profile 1.7 M1.7x0.35 6H" major diameter 1.7678 minor diameter 1.3711 pitch 0.35 angle 60 resizes the face on face at (-0.8707, 0.0871, 11.5667) on bodies 3 in component "hex nut"
component "push rod connector" placed x (1, 0, 0) y (0, 1, 0) z (0, 0, 1) at (0, 0, 0)
component "grub screw" placed x (1, 0, 0) y (0, 1, 0) z (0, 0, 1) at (0, 0, 0)
component "hex nut" placed x (1, 0, 0) y (0, 1, 0) z (0, 0, 1) at (0, 0, 0)
equation "d29 = 1.6 mm / 2"
equation "d32 = 3.9 mm / 2"
